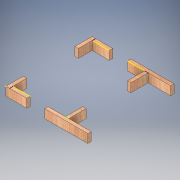
# Autodesk Inventor part: Estructura base
Saved by Autodesk Inventor 2019 (Build 230136000, 136)
## iProperties
Created: 2018-08-15
Part Number: Estructura base
Material: Madera (abedul)
Document SubType Name: Modeling
Designer: Albert Garangou Culebras
Density: 0.55 g/cm^3
Appearance: Abedul - Natural pulido
Mass: 985.875 g
Surface Area: 3092 cm^2
Volume: 1792.5 cm^3
Author: Albert Garangou Culebras
Title: Estructura base
Autodesk Inventor part; units mm, degrees
ref_plane "YZ Plane" through (0, 0, 0) normal (1, 0, 0) x (0, 1, 0)
ref_plane "XZ Plane" through (0, 0, 0) normal (0, 1, 0) x (-1, 0, 0)
ref_plane "XY Plane" through (0, 0, 0) normal (0, 0, 1) x (1, 0, 0)
sketch "Boceto1" plane through (0, 0, 0) normal (0, 1, 0) x (-1, 0, 0)
  line L0 (0, -500) -> (-20, -500)
  line L1 (-20, -500) -> (-20, -400)
  line L2 (-20, -400) -> (0, -400)
  line L3 (0, 0) -> (0, -100)
  line L4 (0, -100) -> (-20, -100)
  line L5 (-20, -100) -> (-20, 0)
  line L6 (-20, 0) -> (0, 0)
  line L7 (-20, 0) -> (-120, 0)
  line L8 (-120, 0) -> (-120, -20)
  line L9 (-120, -20) -> (-20, -20)
  line L10 (-20, -500) -> (-120, -500)
  line L11 (-120, -500) -> (-120, -480)
  line L12 (-120, -480) -> (-20, -480)
  line L13 (-325, 0) -> (-345, 0)
  line L14 (-325, -500) -> (-345, -500)
  line L15 (-325, -480) -> (-225, -480)
  line L16 (-225, -480) -> (-225, -500)
  line L17 (-225, -500) -> (-475, -500)
  line L18 (-475, -500) -> (-475, -480)
  line L19 (-475, -480) -> (-225, -480)
  line L20 (-325, -20) -> (-225, -20)
  line L21 (-225, -20) -> (-225, 0)
  line L22 (-225, 0) -> (-475, 0)
  line L23 (-475, 0) -> (-475, -20)
  line L24 (-475, -20) -> (-225, -20)
  line L25 (-325, -20) -> (-325, -120)
  line L26 (-325, -120) -> (-345, -120)
  line L27 (-345, -120) -> (-345, -20)
  line L28 (0, 0) -> (0, -100)
  line L29 (0, -400) -> (0, -500)
  line L30 (-325, -480) -> (-325, -380)
  line L31 (-325, -380) -> (-345, -380)
  line L32 (-345, -380) -> (-345, -480)
  line L33 (-325, -480) -> (-345, -480)
  dimension "d64" = 100
  dimension "d65" = 20
  constraints: 68 end point, 16 perpendicular, 7 point on line, 6 horizontal, 4 collinear, 3 vertical
  measures "d64" distance of L15.start L30.end
  measures "d65" distance of L30.end L31.end
extrude "Extrusión6" add sketch "Boceto1" along normal blind 50
sketch "Boceto8" plane through (0, 50, 0) normal (0, 1, 0) x (1, 0, 0)
  line L0 (120, 20) -> (20, 20) projected
  line L1 (20, 0) -> (20, 20)
  line L2 (20, 480) -> (120, 480) projected
  line L3 (20, 480) -> (20, 500)
  line L4 (225, 480) -> (325, 480) projected
  line L5 (325, 480) -> (346, 480)
  line L6 (325, 20) -> (346, 20)
  point P0 (0, 0)
  constraints: 8 end point, 2 horizontal, 2 vertical
